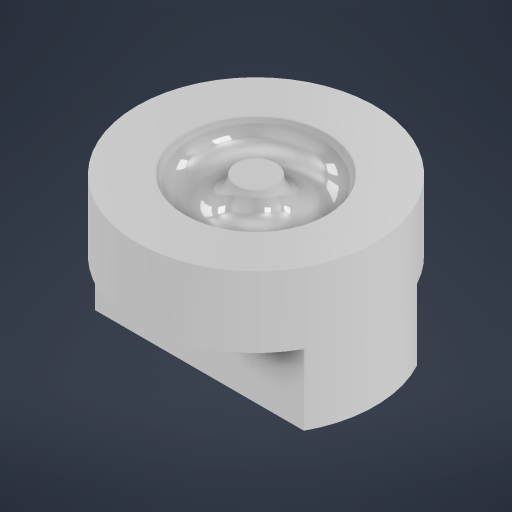
# Autodesk Inventor part: Part1
Saved by Autodesk Inventor 2024 (Build 280153000, 153)
## iProperties
Created: 2023-07-13
Part Number: Part1
Material: Aluminum 6061
Document SubType Name: Modeling
Designer: FER
Density: 2.7 g/cm^3
Appearance: Aluminum - Polished
Author: FER
Autodesk Inventor part; units mm, degrees
ref_plane "YZ Plane" through (0, 0, 0) normal (1, 0, 0) x (0, 1, 0)
ref_plane "XZ Plane" through (0, 0, 0) normal (0, 1, 0) x (-1, 0, 0)
ref_plane "XY Plane" through (0, 0, 0) normal (0, 0, 1) x (1, 0, 0)
sketch "Sketch1" plane through (0, 0, 0) normal (0, 1, 0) x (-1, 0, 0)
  circle A0 centre (0, 0) radius 42
  dimension "d0" = 84
  constraints: 1 centre point, 1 coincident
  measures "d0" diameter of A0
extrude "Extrusion1" add sketch "Sketch1" along normal blind 50
sketch "Sketch3" plane through (0, 0, 0) normal (1, 0, 0) x (0, 1, 0)
  line L0 (50, -42) -> (50, 42) projected
  circle A0 centre (50, -16) radius 9
  line L1 (-11.8, 0) -> (70.8, 0) projected
  line L2 (71.2036, 0) -> (0, 0)
  point P0 (50, -7)
  point P1 (50, -25)
  dimension "d4" = 18
  dimension "d5" = 32
  constraints: 2 end point, 2 point on line, 1 centre point, 1 collinear
  measures "d4" diameter of A0
  measures "d5" diameter of A0.centre L1
revolve "Revolution1" cut sketch "Sketch3" angle 360 about axis through (0, -10, 0) along (0, 1, 0) picked at (45.6277, -15.2948) contours A0 L0
sketch "Sketch4" plane through (0, 0, 0) normal (1, 0, 0) x (0, 1, 0)
  line L0 (0, -42) -> (0, 42) projected
  line L1 (0, -20) -> (25, -20)
  line L2 (25, -20) -> (25, -95.9961)
  line L3 (25, -95.9961) -> (0, -95.9961)
  line L4 (0, -95.9961) -> (0, -20)
  line L5 (-10, 0) -> (60, 0) projected
  line L6 (0, 20) -> (25, 20)
  line L7 (25, 20) -> (25, 95.9961)
  line L8 (25, 95.9961) -> (0, 95.9961)
  line L9 (0, 95.9961) -> (0, 20)
  point P0 (0, 0)
  dimension "d7" = 25
  dimension "d8" = 20
  constraints: 16 end point, 4 symmetric about line, 2 parallel, 1 horizontal, 1 perpendicular, 1 point on line
  measures "d7" distance between parallel lines of L4 L2
  measures "d8" distance between parallel lines of L5 L1
extrude "Extrusion2" cut sketch "Sketch4" along normal mid plane 100
shell "Shell1" thickness 5 removed faces 1 at (11.381, 0, 4.5482)
body "Solid1"
